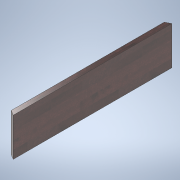
# Autodesk Inventor part: WinchWall-ver1-1111-2021
Saved by Autodesk Inventor 2021 (Build 250183000, 183)
## iProperties
Created: 2021-03-03
Part Number: WinchWall-ver1-1111-2021
Material: Generic
Document SubType Name: Modeling
Designer: CMurray
Density: 1 g/cm^3
Appearance: Wild Cherry - Wild Berries
Author: CMurray
Autodesk Inventor part; units mm, degrees
ref_plane "YZ Plane" through (0, 0, 0) normal (1, 0, 0) x (0, 1, 0)
ref_plane "XZ Plane" through (0, 0, 0) normal (0, 1, 0) x (-1, 0, 0)
ref_plane "XY Plane" through (0, 0, 0) normal (0, 0, 1) x (1, 0, 0)
sketch "Sketch2" plane through (0, 0, 0) normal (0, 1, 0) x (-1, 0, 0)
  line L0 (429.133, 76.1367) -> (429.133, -113.257)
  line L1 (429.133, -113.257) -> (429.133, -791.7227)
  line L2 (429.133, 76.1367) -> (429.133, 732.2867)
  line L3 (378.333, 76.1367) -> (378.333, -88.3086)
  line L4 (378.333, 76.1367) -> (378.333, 762.0047)
  line L5 (378.333, -88.3086) -> (378.333, -817.2173)
  arc A0 (378.333, -817.2173) -> (429.133, -791.7227) centre (0, 0) ccw
  line L6 (429.133, 732.2867) -> (378.333, 762.0047)
  point P0 (429.133, 791.7227)
  dimension "d6" = 429.133
  dimension "d7" = 50.8
  dimension "d10" = 59.436
  constraints: 14 end point, 4 vertical, 2 point on circle, 2 point on line, 1 centre point, 1 coincident
  measures "d6" distance from line of point (0, 0) L0
  measures "d7" distance between parallel lines of L3 L0
  measures "d10" distance of L2.end point (429.133, 791.723)
extrude "Extrusion2" add sketch "Sketch2" along normal blind 381
body "Solid2"
